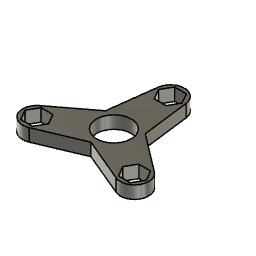
fidget spinner (Autodesk Fusion 360 design; units mm, degrees)
Autodesk Fusion 360 part; units mm, degrees
sketch "Sketch1" plane through (0, 0, 0) normal (0, 0, 1) x (1, 0, 0) in component "fidget spinner"
  circle A0 centre (0, 0) radius 4
  circle A1 centre (0, 0) radius 11
  circle A2 centre (0, 0) radius 13.5
  line L0 (-3.7528, 42.5) -> (-7.5056, 36)
  line L1 (-7.5056, 36) -> (-3.7528, 29.5)
  line L2 (-3.7528, 29.5) -> (3.7528, 29.5)
  line L3 (3.7528, 29.5) -> (7.5056, 36)
  line L4 (7.5056, 36) -> (3.7528, 42.5)
  line L5 (3.7528, 42.5) -> (-3.7528, 42.5)
  line L6 (-12.6841, 7.3232) -> (-8.9294, 37.125)
  line L7 (12.6841, 7.3232) -> (8.9294, 37.125)
  line L8 (-34.9297, -11.5) -> (-38.6825, -18)
  line L9 (-38.6825, -18) -> (-34.9297, -24.5)
  line L10 (-34.9297, -24.5) -> (-27.4241, -24.5)
  line L11 (-27.4241, -24.5) -> (-23.6714, -18)
  line L12 (-23.6714, -18) -> (-27.4241, -11.5)
  line L13 (-27.4241, -11.5) -> (-34.9297, -11.5)
  line L14 (0, -14.6463) -> (-27.6865, -26.2956)
  line L15 (-12.6841, 7.3232) -> (-36.6159, -10.8294)
  line L16 (27.4241, -24.5) -> (34.9297, -24.5)
  line L17 (34.9297, -24.5) -> (38.6825, -18)
  line L18 (38.6825, -18) -> (34.9297, -11.5)
  line L19 (34.9297, -11.5) -> (27.4241, -11.5)
  line L20 (27.4241, -11.5) -> (23.6714, -18)
  line L21 (23.6714, -18) -> (27.4241, -24.5)
  line L22 (12.6841, 7.3232) -> (36.6159, -10.8294)
  line L23 (0, -14.6463) -> (27.6865, -26.2956)
  arc A3 (8.9294, 37.125) -> (-8.9294, 37.125) centre (0, 36) ccw
  arc A4 (-36.6159, -10.8294) -> (-27.6865, -26.2956) centre (-31.1769, -18) ccw
  arc A5 (27.6865, -26.2956) -> (36.6159, -10.8294) centre (31.1769, -18) ccw
  point P0 (0, 36)
  dimension "d1" = 8
  dimension "d2" = 22
  dimension "d3" = 27
  dimension "d4" = 36
  dimension "d5" = 6.5
  dimension "d6" = 18
  constraint coincident A0.centre A1.centre
  constraint concentric A0 A1
  constraint coincident P0 A3.centre
  constraint tangent A2 L6
  constraint tangent L6 A3
  constraint tangent A2 L7
  constraint tangent L7 A3
  measures "d1" diameter of A0
  measures "d2" diameter of A1
  measures "d3" diameter of A2
  measures "d4" distance of A0.centre P0
  measures "d5" distance of P0 L5
  measures "d6" diameter of A3
extrude "Extrude1" add sketch "Sketch1" along normal mid plane 8 contours A2 | L6 L7 L14 L15 L22 L23 A3 A4 A5 in component "fidget spinner"
component "fidget spinner" placed x (1, 0, 0) y (0, 1, 0) z (0, 0, 1) at (0, 0, 0)
